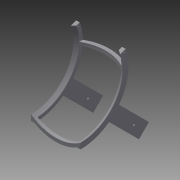
# Autodesk Inventor part: Inner
Saved by Autodesk Inventor 2014 (Build 180170000, 170)
## iProperties
Created: 2014-01-05
Part Number: Inner
Material: Generic
Document SubType Name: Modeling
Designer: Tristan Debrunner
Density: 1 g/cm^3
Appearance: Default
Author: Tristan Debrunner
Autodesk Inventor part; units mm, degrees
ref_plane "YZ Plane" through (0, 0, 0) normal (1, 0, 0) x (0, 1, 0)
ref_plane "XY Plane" through (0, 0, 0) normal (0, 0, 1) x (1, 0, 0)
sketch "Sketch1" plane through (0, 0, 0) normal (0, 0, 1) x (1, 0, 0)
  line L0 (0, 0) -> (0, -41.796)
  line L1 (25.4, -16.396) -> (25.4, -41.796)
  arc A0 (0, 0) -> (25.4, -16.396) centre (177.8, 247.5686) ccw
  line L2 (355.6, 0) -> (355.6, -41.796)
  line L3 (330.2, -16.396) -> (330.2, -41.796)
  arc A1 (330.2, -16.396) -> (355.6, 0) centre (177.8, 247.5686) ccw
  line L4 (0, 304.8) -> (355.6, 304.8)
  line L5 (25.4, -41.796) -> (0, -41.796)
  line L6 (330.2, -41.796) -> (331.8938, -41.796)
  line L7 (331.8938, -41.796) -> (355.6, -41.796)
  constraints: 16 end point, 4 point on circle, 2 centre point, 2 parallel, 2 vertical
revolve "Revolution1" add sketch "Sketch1" angle 110 about axis through (0, 304.8, 0) along (1, 0, 0)
sketch "Sketch2" plane through (0, -41.796, 0) normal (0, 0, 1) x (1, 0, 0)
  line L0 (25.4, 0) -> (25.4, 25.4) projected
  line L1 (355.6, 41.796) -> (355.6, 0) projected
  arc A0 (330.2, 25.4) -> (355.6, 41.796) centre (177.8, 289.3645) ccw projected
  line L2 (330.2, 0) -> (330.2, 25.4) projected
  arc A1 (25.4, 25.4) -> (330.2, 25.4) centre (177.8, 289.3645) ccw
  arc A2 (25.4, 0) -> (330.2, 0) centre (177.8, 263.9645) ccw
  line L3 (25.4, 25.4) -> (25.4, 0)
  line L4 (330.2, 25.4) -> (330.2, 0)
  line L5 (0, 330.2) -> (355.6, 330.2)
  line L6 (355.6, 0) -> (330.2, 0) projected
  dimension "d6" = 304.8
  dimension "d7" = 304.8
  constraints: 6 end point, 4 point on circle, 2 centre point, 2 equal length
  measures "d6" radius of A1
  measures "d7" radius of A2
revolve "Revolution2" add sketch "Sketch2" angle 4 about axis through (0, 288.404, 0) along (1, 0, 0) contours L0 A1 L2 A2
ref_plane "Work Plane1" through (0, 304.8, 0) normal (0, 1, 0) x (-1, 0, 0)
sketch "Sketch3" plane through (0, 304.8, 0) normal (0, 1, 0) x (-1, 0, 0)
  line L0 (-355.6, -346.596) -> (-355.6, -304.8) projected
  line L1 (-330.2, -321.196) -> (-330.2, -346.596) projected
  line L2 (-25.4, -346.596) -> (-25.4, -321.196) projected
  arc A0 (-25.4, -321.196) -> (0, -304.8) centre (-177.8, -57.2314) ccw projected
  line L3 (0, -304.8) -> (0, -346.596) projected
  arc A1 (-330.2, -321.196) -> (-25.4, -321.196) centre (-177.8, -57.2314) ccw
  arc A2 (-330.2, -346.596) -> (-25.4, -346.596) centre (-177.8, -82.6314) ccw
  line L4 (-330.2, -346.596) -> (-330.2, -321.196)
  line L5 (-25.4, -321.196) -> (-25.4, -346.596)
  line L6 (-355.6, 0) -> (0, 0)
  line L7 (-330.2, -346.596) -> (-355.6, -346.596) projected
  arc A3 (-355.6, -304.8) -> (-330.2, -321.196) centre (-177.8, -57.2314) ccw projected
  line L8 (0, -346.596) -> (-25.4, -346.596) projected
  dimension "d11" = 304.8
  dimension "d12" = 304.8
  constraints: 6 end point, 4 point on circle, 2 centre point, 2 collinear
  measures "d11" radius of A1
  measures "d12" radius of A2
revolve "Revolution3" add sketch "Sketch3" angle 4 about axis through (355.6, 304.8, 0) along (-1, 0, 0) contours L1 A1 L2 A2
sketch "Sketch4" plane through (25.4, 304.8, -321.196) normal (1, 0, 0) x (0, 0, -1)
  line L0 (0, 0) -> (25.4, 0) projected
  line L1 (-19.3705, 109.8555) -> (4.4977, 118.5428) projected
  line L2 (-7.4364, 114.1991) -> (-7.4364, 101.4991)
  point P0 (-321.196, -304.8)
  dimension "d15" = 12.7
  constraints: 2 end point, 1 midpoint, 1 perpendicular
  measures "d15" distance of L2.start L2.end
hole "Hole1" at (25.4, 406.2991, -313.7596) direction (1, 0, 0) diameter 6.35 end through all
hole "Hole2" at (25.4, 406.2991, -313.7596) direction (-1, 0, 0) diameter 6.35 end through all
sketch "Sketch5" plane through (0, -41.796, 0) normal (-1, 0, 0) x (0, 0, 1)
  arc A0 (-325.6937, 465.1388) -> (0, 0) centre (0, 346.596) ccw projected
  line L0 (-278.3546, 140.0834) -> (-493.8808, -75.4428)
  line L1 (-493.8808, -75.4428) -> (-422.0387, -147.2848)
  line L2 (-422.0387, -147.2848) -> (-206.5126, 68.2413)
  arc A1 (-278.3546, 140.0834) -> (-206.5126, 68.2413) centre (0, 346.596) ccw
  line L3 (-457.9598, -111.3638) -> (-386.1177, -39.5218)
  circle A2 centre (-386.1177, -39.5218) radius 6.35
  dimension "d36" = 304.8
  dimension "d37" = 101.6
  dimension "d38" = 101.6
  dimension "d39" = 12.7
  constraints: 8 end point, 4 point on circle, 2 centre point, 2 parallel, 1 coincident, 1 concentric, 1 midpoint, 1 perpendicular
  measures "d36" distance of L0.start L0.end
  measures "d37" distance of L0.end L1.end
  measures "d38" distance of L3.start L3.end
  measures "d39" diameter of A2
extrude "Extrusion1" add sketch "Sketch5" against normal blind 25.4
sketch "Sketch6" plane through (355.6, -41.796, 0) normal (1, 0, 0) x (0, 0, -1)
  arc A0 (0, 0) -> (325.6937, 465.1388) centre (0, 346.596) ccw projected
  line L0 (493.8808, -75.4428) -> (278.3546, 140.0834) projected
  line L1 (422.0387, -147.2848) -> (493.8808, -75.4428) projected
  line L2 (206.5126, 68.2413) -> (422.0387, -147.2848) projected
  circle A1 centre (386.1177, -39.5218) radius 6.35 projected
extrude "Extrusion2" add sketch "Sketch6" against normal blind 25.4
body "Solid1"
